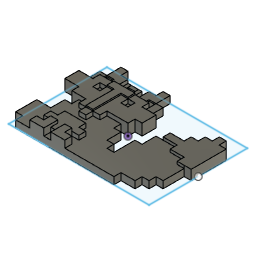
keychain (Autodesk Fusion 360 design; units mm, degrees)
Autodesk Fusion 360 part; units mm, degrees
note: some values were not read from the file. Set by a fixed rule: which sketch regions a step uses.
sketch "base" plane through (0, 0, 0) normal (0, 0, 1) x (1, 0, 0)
  line L0 (50, 0) -> (50, 35)
  line L1 (50, 35) -> (-50, 35)
  line L2 (-50, 35) -> (-50, -35)
  line L3 (-50, -35) -> (50, -35)
  line L4 (50, -35) -> (50, 0)
  dimension "d1" = 50
  dimension "d2" = 35
  dimension "d3" = 100
  dimension "d4" = 70
  dimension "d5" = 100
  dimension "d6" = 35
  constraint perpendicular L0 L1
  constraint perpendicular L1 L2
  constraint perpendicular L2 L3
  constraint perpendicular L1 L4
  measures "d1" distance of origin L0.start
  measures "d2" distance of L0.start L0.end
  measures "d3" distance of L0.end L1.end
  measures "d4" distance of L1.end L2.end
  measures "d5" distance of L2.end L3.end
  measures "d6" distance of L3.end L0.start
extrude "Extrude1" add sketch "base" along normal blind 10 makes body 1
sketch "fox" plane through (0, 0, 10) normal (0, 0, 1) x (-1, 0, 0)
  line L0 (-50, 35) -> (-50, -35)
  line L1 (-50, -35) -> (50, -35)
  line L2 (50, -35) -> (50, 35)
  line L3 (50, 35) -> (-50, 35)
  line L4 (40, -35) -> (40, -30)
  line L5 (45, -15) -> (50, -15)
  line L6 (50, -15) -> (50, -5)
  line L7 (50, -5) -> (40, -5)
  line L8 (40, -5) -> (40, 0)
  line L9 (40, 0) -> (35, 0)
  line L10 (35, 0) -> (35, 5)
  line L11 (35, 5) -> (40, 5)
  line L12 (40, 5) -> (40, 15)
  line L13 (40, 15) -> (50, 15)
  line L14 (50, 15) -> (50, 30)
  line L15 (50, 30) -> (45, 30)
  line L16 (45, 30) -> (45, 35)
  line L17 (45, 35) -> (-25, 35)
  line L18 (40, -35) -> (35, -35)
  line L19 (35, -35) -> (35, -30)
  line L20 (35, -30) -> (30, -30)
  line L21 (30, -30) -> (30, -20)
  line L22 (30, -20) -> (15, -20)
  line L23 (15, -20) -> (15, -25)
  line L24 (10, -35) -> (5, -35)
  line L25 (5, -35) -> (5, -25)
  line L26 (5, -25) -> (0, -25)
  line L27 (0, -25) -> (0, -15)
  line L28 (0, -15) -> (-5, -15)
  line L29 (-5, -15) -> (-5, -5)
  line L30 (-5, -5) -> (0, -5)
  line L31 (0, -5) -> (0, 0)
  line L32 (0, 0) -> (5, 0)
  line L33 (5, 0) -> (5, 5)
  line L34 (5, 5) -> (0, 5)
  line L35 (0, 5) -> (0, 15)
  line L36 (0, 15) -> (-5, 15)
  line L37 (-5, 15) -> (-5, 20)
  line L38 (-5, 20) -> (-10, 20)
  line L39 (-10, 20) -> (-10, 5)
  line L40 (-10, 5) -> (-15, 5)
  line L41 (-15, 5) -> (-15, -5)
  line L42 (-15, -5) -> (-20, -5)
  line L43 (-20, -5) -> (-20, -10)
  line L44 (-20, -10) -> (-30, -10)
  line L45 (-30, -10) -> (-30, -15)
  line L46 (-30, -15) -> (-35, -15)
  line L47 (-35, -15) -> (-35, -20)
  line L48 (-35, -20) -> (-40, -20)
  line L49 (-40, -20) -> (-40, -25)
  line L50 (-40, -25) -> (-45, -25)
  line L51 (-45, -25) -> (-45, -20)
  line L52 (-45, -20) -> (-50, -20)
  line L53 (-50, -20) -> (-50, 5)
  line L54 (-50, 5) -> (-45, 5)
  line L55 (-45, 5) -> (-45, 20)
  line L56 (-45, 20) -> (-40, 20)
  line L57 (-40, 20) -> (-40, 25)
  line L58 (-40, 25) -> (-35, 25)
  line L59 (-35, 25) -> (-35, 30)
  line L60 (-35, 30) -> (-25, 30)
  line L61 (-25, 30) -> (-25, 35)
  line L62 (40, -30) -> (40, -25)
  line L63 (40, -25) -> (45, -25)
  line L64 (45, -25) -> (45, -15)
  line L65 (10, -35) -> (10, -30)
  line L66 (10, -30) -> (15, -30)
  line L67 (15, -30) -> (15, -25)
  dimension "d9" = 5
  dimension "d12" = 5
  dimension "d14" = 10
  dimension "d15" = 10
  dimension "d16" = 5
  dimension "d17" = 5
  dimension "d18" = 5
  dimension "d19" = 5
  dimension "d20" = 10
  dimension "d21" = 10
  dimension "d22" = 15
  dimension "d23" = 5
  dimension "d24" = 5
  dimension "d25" = 70
  dimension "d26" = 5
  dimension "d27" = 5
  dimension "d28" = 5
  dimension "d29" = 10
  dimension "d30" = 15
  dimension "d31" = 5
  dimension "d34" = 5
  dimension "d35" = 10
  dimension "d36" = 5
  dimension "d37" = 10
  dimension "d38" = 5
  dimension "d39" = 10
  dimension "d40" = 5
  dimension "d41" = 5
  dimension "d42" = 5
  dimension "d43" = 5
  dimension "d44" = 5
  dimension "d45" = 10
  dimension "d46" = 5
  dimension "d47" = 5
  dimension "d48" = 5
  dimension "d49" = 15
  dimension "d50" = 5
  dimension "d51" = 10
  dimension "d52" = 5
  dimension "d53" = 5
  dimension "d54" = 10
  dimension "d55" = 5
  dimension "d56" = 5
  dimension "d57" = 5
  dimension "d58" = 5
  dimension "d59" = 5
  dimension "d60" = 5
  dimension "d61" = 5
  dimension "d62" = 5
  dimension "d63" = 25
  dimension "d64" = 5
  dimension "d65" = 15
  dimension "d66" = 5
  dimension "d67" = 5
  dimension "d68" = 5
  dimension "d69" = 5
  dimension "d70" = 10
  dimension "d71" = 5
  dimension "d78" = 5
  dimension "d79" = 5
  dimension "d152" = 5
  dimension "d153" = 5
  dimension "d154" = 5
  constraint coincident L1 L4.start
  constraint perpendicular L2 L5
  constraint perpendicular L5 L6
  constraint perpendicular L6 L7
  constraint perpendicular L7 L8
  constraint perpendicular L6 L9
  constraint perpendicular L9 L10
  constraint perpendicular L2 L11
  constraint perpendicular L7 L12
  constraint perpendicular L2 L13
  constraint perpendicular L13 L14
  constraint perpendicular L14 L15
  constraint perpendicular L3 L16
  constraint coincident L3 L17.end
  constraint perpendicular L16 L17
  constraint perpendicular L4 L18
  constraint perpendicular L18 L19
  constraint perpendicular L4 L20
  constraint perpendicular L18 L21
  constraint perpendicular L0 L22
  constraint perpendicular L22 L23
  constraint perpendicular L24 L25
  constraint perpendicular L25 L26
  constraint perpendicular L24 L27
  constraint perpendicular L27 L28
  constraint perpendicular L28 L29
  constraint perpendicular L23 L30
  constraint perpendicular L28 L31
  constraint perpendicular L23 L32
  constraint perpendicular L32 L33
  constraint perpendicular L33 L34
  constraint perpendicular L34 L35
  constraint perpendicular L35 L36
  constraint perpendicular L36 L37
  constraint perpendicular L37 L38
  constraint perpendicular L36 L39
  constraint perpendicular L39 L40
  constraint perpendicular L40 L41
  constraint perpendicular L41 L42
  constraint perpendicular L42 L43
  constraint perpendicular L41 L44
  constraint perpendicular L44 L45
  constraint perpendicular L25 L46
  constraint perpendicular L44 L47
  constraint perpendicular L25 L48
  constraint perpendicular L44 L49
  constraint perpendicular L25 L50
  constraint perpendicular L44 L51
  constraint perpendicular L0 L52
  constraint perpendicular L52 L53
  constraint perpendicular L53 L54
  constraint perpendicular L54 L55
  constraint perpendicular L55 L56
  constraint perpendicular L56 L57
  constraint perpendicular L55 L58
  constraint perpendicular L58 L59
  constraint perpendicular L55 L60
  constraint perpendicular L17 L61
  constraint parallel L4 L62
  constraint perpendicular L62 L63
  constraint perpendicular L5 L64
  constraint perpendicular L1 L65
  constraint perpendicular L65 L66
  constraint perpendicular L1 L67
  measures "d9" distance of L4.start L4.end
  measures "d12" distance of L5.start L5.end
  measures "d14" distance of L5.end L6.end
  measures "d15" distance of L6.end L7.end
  measures "d16" distance of L7.end L8.end
  measures "d17" distance of L8.end L9.end
  measures "d18" distance of L9.end L10.end
  measures "d19" distance of L10.end L11.end
  measures "d20" distance of L11.end L12.end
  measures "d21" distance of L12.end L13.end
  measures "d22" distance of L13.end L14.end
  measures "d23" distance of L14.end L15.end
  measures "d24" distance of L15.end L16.end
  measures "d25" distance of L16.end L17.end
  measures "d26" distance of L4.start L18.end
  measures "d27" distance of L18.end L19.end
  measures "d28" distance of L19.end L20.end
  measures "d29" distance of L20.end L21.end
  measures "d30" distance of L21.end L22.end
  measures "d31" distance of L22.end L23.end
  measures "d34" distance of L24.start L24.end
  measures "d35" distance of L24.end L25.end
  measures "d36" distance of L25.end L26.end
  measures "d37" distance of L26.end L27.end
  measures "d38" distance of L27.end L28.end
  measures "d39" distance of L28.end L29.end
  measures "d40" distance of L29.end L30.end
  measures "d41" distance of L30.end L31.end
  measures "d42" distance of L31.end L32.end
  measures "d43" distance of L32.end L33.end
  measures "d44" distance of L33.end L34.end
  measures "d45" distance of L34.end L35.end
  measures "d46" distance of L35.end L36.end
  measures "d47" distance of L36.end L37.end
  measures "d48" distance of L37.end L38.end
  measures "d49" distance of L38.end L39.end
  measures "d50" distance of L39.end L40.end
  measures "d51" distance of L40.end L41.end
  measures "d52" distance of L41.end L42.end
  measures "d53" distance of L42.end L43.end
  measures "d54" distance of L43.end L44.end
  measures "d55" distance of L44.end L45.end
  measures "d56" distance of L45.end L46.end
  measures "d57" distance of L46.end L47.end
  measures "d58" distance of L47.end L48.end
  measures "d59" distance of L48.end L49.end
  measures "d60" distance of L49.end L50.end
  measures "d61" distance of L50.end L51.end
  measures "d62" distance of L51.end L52.end
  measures "d63" distance of L52.end L53.end
  measures "d64" distance of L53.end L54.end
  measures "d65" distance of L54.end L55.end
  measures "d66" distance of L55.end L56.end
  measures "d67" distance of L56.end L57.end
  measures "d68" distance of L57.end L58.end
  measures "d69" distance of L58.end L59.end
  measures "d70" distance of L59.end L60.end
  measures "d71" distance of L60.end L17.end
  measures "d78" distance of L4.end L62.end
  measures "d79" distance of L62.end L63.end
  measures "d152" distance of L24.start L65.end
  measures "d153" distance of L65.end L66.end
  measures "d154" distance of L66.end L23.end
extrude "Extrude2" cut sketch "fox" against normal blind 0.1 contours L0 L1 L2 L3 L4 L5 L6 L7 L8 L9 L10 L11 L12 L13 L14 L15 L16 L17 L18 L19 L20 L21 L22 L23 L24 L25 L26 L27 L28 L29 L30 L31 L32 L33 L34 L35 L36 L37 L38 L39 L40 L41 L42 L43 L44 L45 L46 L47 L48 L49 L50 L51 L52 L53 L54 L55 L56 L57 L58 L59 L60 L61 L62 L63 L64 L65 L66 L67 bodies 1
extrude "Extrude3" add 1 faces at (-18.3333, 6.6667, 9.9) along direction (0, 0, 1) blind 0.1 on bodies 1 bodies 1
extrude "Extrude4" cut sketch "fox" against normal blind 10 contours L0 L3 L54 L55 L56 L57 L58 L59 L60 L61 | L0 L1 L25 L26 L27 L28 L29 L30 L31 L32 L33 L34 L35 L36 L37 L38 L39 L40 L41 L42 L43 L44 L45 L46 L47 L48 L49 L50 L51 L52 | L2 L3 L15 L16 | L1 L19 L20 L21 L22 L23 L65 L66 L67 | L2 L7 L8 L9 L10 L11 L12 L13 | L1 L2 L4 L5 L62 L63 L64 bodies 1
sketch "ears" plane through (0, 0, 10) normal (0, 0, 1) x (-1, 0, 0)
  line L0 (-45, 5) -> (-50, 5)
  line L1 (-50, 5) -> (-50, -20)
  line L2 (-50, -20) -> (-45, -20)
  line L3 (-45, -20) -> (-45, -25)
  line L4 (-45, -25) -> (-40, -25)
  line L5 (-40, -25) -> (-40, -20)
  line L6 (-40, -20) -> (-35, -20)
  line L7 (-35, -20) -> (-35, -15)
  line L8 (-35, -15) -> (-30, -15)
  line L9 (-30, -15) -> (-30, -10)
  line L10 (-30, -10) -> (-20, -10)
  line L11 (-20, -10) -> (-20, -5)
  line L12 (-20, -5) -> (-15, -5)
  line L13 (-15, -5) -> (-15, 5)
  line L14 (-15, 5) -> (-10, 5)
  line L15 (-10, 5) -> (-10, 20)
  line L16 (-10, 20) -> (-5, 20)
  line L17 (-5, 20) -> (-5, 15)
  line L18 (-5, 15) -> (0, 15)
  line L19 (0, 15) -> (0, 5)
  line L20 (0, 5) -> (5, 5)
  line L21 (5, 5) -> (5, 0)
  line L22 (5, 0) -> (0, 0)
  line L23 (0, 0) -> (0, -5)
  line L24 (0, -5) -> (-5, -5)
  line L25 (-5, -5) -> (-5, -15)
  line L26 (-5, -15) -> (0, -15)
  line L27 (0, -15) -> (0, -25)
  line L28 (0, -25) -> (5, -25)
  line L29 (5, -25) -> (5, -35)
  line L30 (5, -35) -> (10, -35)
  line L31 (40, -35) -> (40, -25)
  line L32 (45, -15) -> (50, -15)
  line L33 (50, -15) -> (50, -5)
  line L34 (50, -5) -> (40, -5)
  line L35 (40, -5) -> (40, 0)
  line L36 (40, 0) -> (35, 0)
  line L37 (35, 0) -> (35, 5)
  line L38 (35, 5) -> (40, 5)
  line L39 (40, 5) -> (40, 15)
  line L40 (40, 15) -> (50, 15)
  line L41 (50, 15) -> (50, 30)
  line L42 (50, 30) -> (45, 30)
  line L43 (45, 30) -> (45, 35)
  line L44 (45, 35) -> (-25, 35)
  line L45 (-25, 35) -> (-25, 30)
  line L46 (-25, 30) -> (-35, 30)
  line L47 (-35, 30) -> (-35, 25)
  line L48 (-35, 25) -> (-40, 25)
  line L49 (-40, 25) -> (-40, 20)
  line L50 (-40, 20) -> (-45, 20)
  line L51 (-45, 20) -> (-45, 5)
  line L52 (40, -25) -> (45, -25)
  line L53 (45, -25) -> (45, -15)
  line L54 (40, -25) -> (35, -25)
  line L55 (35, -25) -> (35, -20)
  line L56 (35, -20) -> (40, -20)
  line L57 (40, -20) -> (40, -25)
  line L58 (10, -25) -> (5, -25)
  line L59 (5, -25) -> (5, -20)
  line L60 (5, -20) -> (10, -20)
  line L61 (10, -20) -> (10, -25)
  line L62 (10, -35) -> (10, -30)
  line L63 (10, -30) -> (15, -30)
  line L64 (15, -30) -> (15, -20)
  line L65 (15, -20) -> (30, -20)
  line L66 (30, -20) -> (30, -30)
  line L67 (30, -30) -> (35, -30)
  line L68 (35, -30) -> (35, -35)
  line L69 (35, -35) -> (40, -35)
  dimension "d80" = 5
  dimension "d81" = 5
  dimension "d82" = 5
  dimension "d83" = 5
  dimension "d84" = 5
  dimension "d85" = 5
  dimension "d86" = 5
  dimension "d87" = 5
  constraint coincident L31.end L52.start
  constraint perpendicular L31 L54
  constraint perpendicular L52 L55
  constraint perpendicular L31 L56
  constraint perpendicular L52 L57
  constraint perpendicular L28 L59
  constraint perpendicular L29 L60
  constraint perpendicular L58 L61
  measures "d80" distance of L31.end L54.end
  measures "d81" distance of L54.end L55.end
  measures "d82" distance of L55.end L56.end
  measures "d83" distance of L56.end L31.end
  measures "d84" distance of L58.start L28.end
  measures "d85" distance of L28.end L59.end
  measures "d86" distance of L59.end L60.end
  measures "d87" distance of L60.end L58.start
sketch "eyes" plane through (0, 0, 10) normal (0, 0, 1) x (-1, 0, 0)
  line L0 (35, -15) -> (30, -15)
  line L1 (30, -15) -> (30, -10)
  line L2 (30, -10) -> (35, -10)
  line L3 (35, -10) -> (35, -15)
  line L4 (15, -15) -> (10, -15)
  line L5 (10, -15) -> (10, -10)
  line L6 (10, -10) -> (15, -10)
  line L7 (15, -10) -> (15, -15)
  dimension "d88" = 5
  dimension "d89" = 5
  dimension "d90" = 5
  dimension "d91" = 5
  dimension "d92" = 5
  dimension "d93" = 5
  dimension "d94" = 5
  dimension "d95" = 5
  constraint horizontal L0
  constraint perpendicular L0 L1
  constraint perpendicular L1 L2
  constraint perpendicular L2 L3
  constraint perpendicular L1 L4
  constraint perpendicular L0 L5
  constraint perpendicular L1 L6
  constraint perpendicular L0 L7
  measures "d88" distance of L0.start L0.end
  measures "d89" distance of L0.end L1.end
  measures "d90" distance of L1.end L2.end
  measures "d91" distance of L2.end L0.start
  measures "d92" distance of L4.start L4.end
  measures "d93" distance of L4.end L5.end
  measures "d94" distance of L5.end L6.end
  measures "d95" distance of L6.end L4.start
sketch "face" plane through (0, 0, 10) normal (0, 0, 1) x (-1, 0, 0)
  line L0 (35, 0) -> (30, 0)
  line L1 (30, 0) -> (30, 5)
  line L2 (30, 5) -> (25, 5)
  line L3 (20, 5) -> (15, 5)
  line L4 (15, 5) -> (15, 0)
  line L5 (15, 0) -> (10, 0)
  line L6 (10, 0) -> (0, 0)
  line L7 (0, 0) -> (0, -5)
  line L8 (0, -5) -> (-5, -5)
  line L9 (-5, -5) -> (-5, -15)
  line L10 (-5, -15) -> (5, -15)
  line L11 (5, -15) -> (5, -20)
  line L12 (5, -20) -> (10, -20)
  line L13 (10, -20) -> (15, -20)
  line L14 (15, -20) -> (15, -15)
  line L15 (30, -15) -> (30, -20)
  line L16 (30, -20) -> (40, -20)
  line L17 (40, -20) -> (40, -15)
  line L18 (40, -15) -> (50, -15)
  line L19 (50, -15) -> (50, -5)
  line L20 (50, -5) -> (40, -5)
  line L21 (40, -5) -> (40, 0)
  line L22 (40, 0) -> (35, 0)
  line L23 (30, -15) -> (25, -15)
  line L24 (25, -15) -> (25, 5)
  line L25 (15, -15) -> (20, -15)
  line L26 (20, -15) -> (20, 5)
  dimension "d96" = 5
  dimension "d97" = 5
  dimension "d98" = 5
  dimension "d102" = 5
  dimension "d103" = 5
  dimension "d104" = 5
  dimension "d105" = 10
  dimension "d106" = 5
  dimension "d107" = 5
  dimension "d108" = 10
  dimension "d109" = 5
  dimension "d110" = 5
  dimension "d111" = 5
  dimension "d112" = 5
  dimension "d113" = 5
  dimension "d114" = 10
  dimension "d115" = 5
  dimension "d116" = 10
  dimension "d117" = 10
  dimension "d118" = 10
  dimension "d119" = 5
  dimension "d120" = 5
  dimension "d121" = 5
  dimension "d122" = 20
  dimension "d123" = 5
  dimension "d124" = 20
  constraint horizontal L0
  constraint perpendicular L0 L1
  constraint perpendicular L1 L2
  constraint perpendicular L3 L4
  constraint perpendicular L4 L5
  constraint parallel L5 L6
  constraint perpendicular L5 L7
  constraint perpendicular L7 L8
  constraint perpendicular L5 L9
  constraint perpendicular L9 L10
  constraint perpendicular L10 L11
  constraint perpendicular L9 L12
  constraint parallel L12 L13
  constraint perpendicular L12 L14
  constraint perpendicular L12 L15
  constraint perpendicular L15 L16
  constraint perpendicular L12 L17
  constraint perpendicular L17 L18
  constraint perpendicular L12 L19
  constraint perpendicular L19 L20
  constraint perpendicular L12 L21
  constraint perpendicular L21 L22
  constraint perpendicular L15 L23
  constraint perpendicular L2 L24
  constraint perpendicular L14 L25
  constraint perpendicular L25 L26
  measures "d96" distance of L0.start L0.end
  measures "d97" distance of L0.end L1.end
  measures "d98" distance of L1.end L2.end
  measures "d102" distance of L3.start L3.end
  measures "d103" distance of L3.end L4.end
  measures "d104" distance of L4.end L5.end
  measures "d105" distance of L5.end L6.end
  measures "d106" distance of L6.end L7.end
  measures "d107" distance of L7.end L8.end
  measures "d108" distance of L9.end L10.end
  measures "d109" distance of L10.end L11.end
  measures "d110" distance of L11.end L12.end
  measures "d111" distance of L12.end L13.end
  measures "d112" distance of L13.end L14.end
  measures "d113" distance of L15.start L15.end
  measures "d114" distance of L15.end L16.end
  measures "d115" distance of L16.end L17.end
  measures "d116" distance of L17.end L18.end
  measures "d117" distance of L18.end L19.end
  measures "d118" distance of L19.end L20.end
  measures "d119" distance of L20.end L21.end
  measures "d120" distance of L21.end L0.start
  measures "d121" distance of L15.start L23.end
  measures "d122" distance of L23.end L2.end
  measures "d123" distance of L14.end L25.end
  measures "d124" distance of L25.end L3.start
sketch "nose" plane through (0, 0, 10) normal (0, 0, 1) x (-1, 0, 0)
  line L0 (25, 5) -> (20, 5)
  line L1 (20, 5) -> (20, 10)
  line L2 (20, 10) -> (25, 10)
  line L3 (25, 10) -> (25, 5)
  dimension "d125" = 5
  dimension "d126" = 5
  constraint horizontal L0
  constraint vertical L1
  constraint horizontal L2
  constraint vertical L3
  measures "d125" distance of L0.start L0.end
  measures "d126" distance of L0.start L2.end
sketch "chest" plane through (0, 0, 10) normal (0, 0, 1) x (-1, 0, 0)
  line L0 (25, 30) -> (20, 30)
  line L1 (20, 30) -> (20, 25)
  line L2 (20, 25) -> (10, 25)
  line L3 (10, 25) -> (10, 20)
  line L4 (10, 20) -> (15, 20)
  line L5 (15, 20) -> (15, 15)
  line L6 (15, 15) -> (30, 15)
  line L7 (30, 15) -> (30, 20)
  line L8 (30, 20) -> (35, 20)
  line L9 (35, 20) -> (35, 25)
  line L10 (35, 25) -> (25, 25)
  line L11 (25, 25) -> (25, 30)
  dimension "d127" = 5
  dimension "d128" = 5
  dimension "d129" = 10
  dimension "d130" = 5
  dimension "d131" = 5
  dimension "d132" = 5
  dimension "d133" = 15
  dimension "d134" = 5
  dimension "d135" = 5
  dimension "d136" = 5
  dimension "d137" = 10
  dimension "d138" = 5
  constraint horizontal L0
  constraint perpendicular L0 L1
  constraint perpendicular L1 L2
  constraint perpendicular L2 L3
  constraint perpendicular L3 L4
  constraint perpendicular L4 L5
  constraint perpendicular L5 L6
  constraint perpendicular L6 L7
  constraint perpendicular L5 L8
  constraint perpendicular L6 L9
  constraint perpendicular L5 L10
  constraint perpendicular L10 L11
  measures "d127" distance of L0.start L0.end
  measures "d128" distance of L0.end L1.end
  measures "d129" distance of L1.end L2.end
  measures "d130" distance of L2.end L3.end
  measures "d131" distance of L3.end L4.end
  measures "d132" distance of L4.end L5.end
  measures "d133" distance of L5.end L6.end
  measures "d134" distance of L6.end L7.end
  measures "d135" distance of L7.end L8.end
  measures "d136" distance of L8.end L9.end
  measures "d137" distance of L9.end L10.end
  measures "d138" distance of L10.end L0.start
sketch "legs" plane through (0, 0, 10) normal (0, 0, 1) x (-1, 0, 0)
  line L0 (25, 30) -> (25, 35)
  line L1 (25, 35) -> (35, 35)
  line L2 (35, 35) -> (35, 30)
  line L3 (35, 30) -> (30, 30)
  line L4 (30, 30) -> (30, 25)
  line L5 (30, 25) -> (25, 25)
  line L6 (25, 25) -> (25, 30)
  line L7 (20, 25) -> (20, 35)
  line L8 (20, 35) -> (10, 35)
  line L9 (10, 35) -> (10, 30)
  line L10 (10, 30) -> (15, 30)
  line L11 (15, 30) -> (15, 25)
  line L12 (15, 25) -> (20, 25)
  dimension "d139" = 5
  dimension "d140" = 10
  dimension "d141" = 5
  dimension "d142" = 5
  dimension "d143" = 5
  dimension "d144" = 5
  dimension "d145" = 5
  dimension "d146" = 10
  dimension "d147" = 10
  dimension "d148" = 5
  dimension "d149" = 5
  dimension "d150" = 5
  dimension "d151" = 5
  constraint vertical L0
  constraint perpendicular L0 L1
  constraint perpendicular L1 L2
  constraint perpendicular L2 L3
  constraint perpendicular L3 L4
  constraint perpendicular L4 L5
  constraint perpendicular L5 L6
  constraint vertical L7
  constraint perpendicular L7 L8
  constraint perpendicular L8 L9
  constraint perpendicular L9 L10
  constraint perpendicular L10 L11
  constraint perpendicular L11 L12
  measures "d139" distance of L0.start L0.end
  measures "d140" distance of L0.end L1.end
  measures "d141" distance of L1.end L2.end
  measures "d142" distance of L2.end L3.end
  measures "d143" distance of L3.end L4.end
  measures "d144" distance of L4.end L5.end
  measures "d145" distance of L5.end L0.start
  measures "d146" distance of L7.start L7.end
  measures "d147" distance of L7.end L8.end
  measures "d148" distance of L8.end L9.end
  measures "d149" distance of L9.end L10.end
  measures "d150" distance of L10.end L11.end
  measures "d151" distance of L11.end L7.start
sketch "tail" plane through (0, 0, 10) normal (0, 0, 1) x (-1, 0, 0)
  line L0 (-45, 5) -> (-50, 5)
  line L1 (-50, 5) -> (-50, -20)
  line L2 (-50, -20) -> (-45, -20)
  line L3 (-45, -20) -> (-45, -25)
  line L4 (-45, -25) -> (-40, -25)
  line L5 (-40, -25) -> (-40, -20)
  line L6 (-40, -20) -> (-35, -20)
  line L7 (-35, -20) -> (-35, -15)
  line L8 (-35, -15) -> (-30, -15)
  line L9 (-30, -15) -> (-30, -10)
  line L10 (-30, -10) -> (-25, -10)
  line L11 (-25, -10) -> (-20, -10)
  line L12 (-20, -10) -> (-20, -5)
  line L13 (-20, -5) -> (-25, -5)
  line L14 (-25, -5) -> (-30, -5)
  line L15 (-30, -5) -> (-30, 0)
  line L16 (-30, 0) -> (-40, 0)
  line L17 (-40, 0) -> (-40, 5)
  line L18 (-40, 5) -> (-45, 5)
  dimension "d162" = 5
  dimension "d163" = 25
  dimension "d164" = 5
  dimension "d165" = 5
  dimension "d166" = 5
  dimension "d167" = 5
  dimension "d168" = 5
  dimension "d169" = 5
  dimension "d170" = 5
  dimension "d173" = 5
  dimension "d174" = 5
  dimension "d175" = 5
  dimension "d176" = 5
  dimension "d177" = 5
  dimension "d178" = 5
  dimension "d179" = 10
  dimension "d180" = 5
  dimension "d181" = 5
  constraint perpendicular L0 L1
  constraint perpendicular L1 L2
  constraint perpendicular L2 L3
  constraint perpendicular L1 L4
  constraint perpendicular L4 L5
  constraint perpendicular L1 L6
  constraint perpendicular L6 L7
  constraint perpendicular L1 L8
  constraint perpendicular L8 L9
  constraint perpendicular L9 L10
  constraint perpendicular L9 L11
  constraint perpendicular L10 L12
  constraint perpendicular L9 L13
  constraint perpendicular L9 L14
  constraint perpendicular L10 L15
  constraint perpendicular L9 L16
  constraint perpendicular L10 L17
  constraint perpendicular L9 L18
  measures "d162" distance of L0.start L0.end
  measures "d163" distance of L0.end L1.end
  measures "d164" distance of L1.end L2.end
  measures "d165" distance of L2.end L3.end
  measures "d166" distance of L3.end L4.end
  measures "d167" distance of L5.end L6.end
  measures "d168" distance of L6.end L7.end
  measures "d169" distance of L7.end L8.end
  measures "d170" distance of L8.end L9.end
  measures "d173" distance of L9.end L10.end
  measures "d174" distance of L10.end L11.end
  measures "d175" distance of L11.end L12.end
  measures "d176" distance of L12.end L13.end
  measures "d177" distance of L13.end L14.end
  measures "d178" distance of L14.end L15.end
  measures "d179" distance of L15.end L16.end
  measures "d180" distance of L16.end L17.end
  measures "d181" distance of L17.end L0.start
extrude "Extrude5" cut sketch "chest" against normal blind 1 bodies 1
extrude "Extrude6" cut sketch "face" against normal blind 2 bodies 1
extrude "Extrude7" cut sketch "eyes" sketch "ears" against normal blind 5 of sketch 2 contours L58 L59 L60 L61 | L54 L55 L56 L57 bodies 1
extrude "Extrude8" cut sketch "nose" against normal blind 5 bodies 1
extrude "Extrude9" cut sketch "tail" against normal blind 2 bodies 1
sketch "contour " plane through (0, 0, 10) normal (0, 0, 1) x (-1, 0, 0)
  line L0 (-45, 5) -> (-45, 20)
  line L1 (-45, 20) -> (-40, 20)
  line L2 (-40, 20) -> (-40, 25)
  line L3 (-40, 25) -> (-35, 25)
  line L4 (-35, 25) -> (-35, 30)
  line L5 (-35, 30) -> (-25, 30)
  line L6 (-25, 30) -> (-25, 35)
  line L7 (-25, 35) -> (10, 35)
  line L8 (10, 35) -> (10, 30)
  line L9 (10, 30) -> (15, 30)
  line L10 (15, 30) -> (15, 25)
  line L11 (15, 25) -> (10, 25)
  line L12 (10, 25) -> (10, 20)
  line L13 (10, 20) -> (15, 20)
  line L14 (15, 20) -> (15, 15)
  line L15 (15, 15) -> (30, 15)
  line L16 (30, 15) -> (30, 20)
  line L17 (30, 20) -> (35, 20)
  line L18 (35, 20) -> (35, 25)
  line L19 (35, 25) -> (30, 25)
  line L20 (30, 25) -> (30, 30)
  line L21 (30, 30) -> (35, 30)
  line L22 (35, 30) -> (35, 35)
  line L23 (35, 35) -> (45, 35)
  line L24 (45, 35) -> (45, 30)
  line L25 (45, 30) -> (50, 30)
  line L26 (50, 30) -> (50, 15)
  line L27 (50, 15) -> (40, 15)
  line L28 (40, 15) -> (40, 5)
  line L29 (40, 5) -> (35, 5)
  line L30 (35, 5) -> (35, 0)
  line L31 (35, 0) -> (30, 0)
  line L32 (30, 0) -> (30, 5)
  line L33 (30, 5) -> (25, 5)
  line L34 (25, 5) -> (25, 10)
  line L35 (25, 10) -> (20, 10)
  line L36 (20, 10) -> (20, 5)
  line L37 (20, 5) -> (15, 5)
  line L38 (15, 5) -> (15, 0)
  line L39 (15, 0) -> (5, 0)
  line L40 (5, 0) -> (5, 5)
  line L41 (5, 5) -> (0, 5)
  line L42 (0, 5) -> (0, 15)
  line L43 (0, 15) -> (-5, 15)
  line L44 (-5, 15) -> (-5, 20)
  line L45 (-5, 20) -> (-10, 20)
  line L46 (-10, 20) -> (-10, 5)
  line L47 (-10, 5) -> (-15, 5)
  line L48 (-15, 5) -> (-15, -5)
  line L49 (-15, -5) -> (-30, -5)
  line L50 (-30, -5) -> (-30, 0)
  line L51 (-30, 0) -> (-40, 0)
  line L52 (-40, 0) -> (-40, 5)
  line L53 (-40, 5) -> (-45, 5)
  line L54 (45, -15) -> (40, -15)
  line L55 (40, -15) -> (40, -25)
  line L56 (40, -25) -> (45, -25)
  line L57 (45, -25) -> (45, -15)
  line L58 (30, -20) -> (30, -30)
  line L59 (30, -30) -> (35, -30)
  line L60 (35, -30) -> (35, -35)
  line L61 (35, -35) -> (40, -35)
  line L62 (40, -35) -> (40, -25)
  line L63 (35, -25) -> (40, -25)
  line L64 (35, -25) -> (35, -20)
  line L65 (35, -20) -> (30, -20)
  line L66 (15, -20) -> (10, -20)
  line L67 (10, -20) -> (10, -25)
  line L68 (10, -25) -> (5, -25)
  line L69 (5, -25) -> (5, -35)
  line L70 (5, -35) -> (10, -35)
  line L71 (10, -35) -> (10, -30)
  line L72 (10, -30) -> (15, -30)
  line L73 (15, -30) -> (15, -20)
  line L74 (5, -25) -> (0, -25)
  line L75 (0, -25) -> (0, -15)
  line L76 (0, -15) -> (5, -15)
  line L77 (5, -15) -> (5, -25)
  line L78 (25, 30) -> (20, 30)
  line L79 (20, 30) -> (20, 35)
  line L80 (20, 35) -> (25, 35)
  line L81 (25, 35) -> (25, 30)
  dimension "d192" = 15
  constraint vertical L0
  constraint perpendicular L0 L1
  constraint perpendicular L1 L2
  constraint perpendicular L2 L3
  constraint perpendicular L3 L4
  constraint perpendicular L4 L5
  constraint perpendicular L5 L6
  constraint perpendicular L6 L7
  constraint perpendicular L7 L8
  constraint perpendicular L8 L9
  constraint perpendicular L9 L10
  constraint perpendicular L10 L11
  constraint perpendicular L11 L12
  constraint perpendicular L12 L13
  constraint perpendicular L13 L14
  constraint perpendicular L14 L15
  constraint perpendicular L15 L16
  constraint perpendicular L16 L17
  constraint perpendicular L17 L18
  constraint perpendicular L18 L19
  constraint perpendicular L17 L20
  constraint perpendicular L18 L21
  constraint perpendicular L17 L22
  constraint perpendicular L22 L23
  constraint perpendicular L23 L24
  constraint perpendicular L24 L25
  constraint perpendicular L25 L26
  constraint perpendicular L26 L27
  constraint perpendicular L27 L28
  constraint perpendicular L26 L29
  constraint perpendicular L29 L30
  constraint perpendicular L30 L31
  constraint perpendicular L29 L32
  constraint perpendicular L32 L33
  constraint perpendicular L33 L34
  constraint perpendicular L34 L35
  constraint perpendicular L35 L36
  constraint perpendicular L36 L37
  constraint perpendicular L37 L38
  constraint perpendicular L38 L39
  constraint perpendicular L39 L40
  constraint perpendicular L40 L41
  constraint perpendicular L41 L42
  constraint perpendicular L42 L43
  constraint perpendicular L43 L44
  constraint perpendicular L44 L45
  constraint perpendicular L45 L46
  constraint perpendicular L44 L47
  constraint perpendicular L45 L48
  constraint perpendicular L48 L49
  constraint perpendicular L49 L50
  constraint perpendicular L50 L51
  constraint perpendicular L51 L52
  constraint horizontal L54
  constraint perpendicular L54 L55
  constraint perpendicular L55 L56
  constraint perpendicular L54 L57
  constraint perpendicular L54 L58
  constraint perpendicular L58 L59
  constraint perpendicular L59 L60
  constraint perpendicular L60 L61
  constraint perpendicular L56 L62
  constraint perpendicular L62 L63
  constraint perpendicular L63 L64
  constraint perpendicular L58 L65
  constraint horizontal L66
  constraint perpendicular L66 L67
  constraint perpendicular L67 L68
  constraint perpendicular L66 L69
  constraint perpendicular L69 L70
  constraint perpendicular L70 L71
  constraint perpendicular L71 L72
  constraint perpendicular L66 L73
  constraint perpendicular L69 L74
  constraint perpendicular L74 L75
  constraint perpendicular L75 L76
  constraint perpendicular L68 L77
  constraint horizontal L78
  constraint vertical L79
  constraint horizontal L80
  constraint vertical L81
  measures "d192" distance of L0.start L0.end
extrude "Extrude10" add sketch "eyes" sketch "ears" against normal blind 4 separate body of sketch 2 contours L58 L59 L60 L61 | L54 L55 L56 L57 makes body 2 at (-6.6667, 21.6667, 10) makes body 3 at (-33.3333, 13.3333, 10) makes body 4 at (-13.3333, 13.3333, 10) makes body 5 at (-38.3333, 23.3333, 10)
extrude "Extrude11" cut 4 faces at (-33.3333, 13.3333, 10) (-13.3333, 13.3333, 10) (-6.6667, 21.6667, 10) (-38.3333, 23.3333, 10) along direction (0, 0, -1) blind 3 on bodies 2 3 4 5 bodies 2 3 4 5
extrude "Extrude12" cut sketch "legs" against normal blind 9 bodies 1
extrude "Extrude13" add 1 faces at (-23.3333, -6.6667, 5) along direction (0, 0, 1) blind 4 on bodies 1 bodies 1
extrude "Extrude14" cut sketch "contour " against normal blind 5 bodies 1
extrude "Extrude15" add 2 faces at (-26.6667, -30, 1) (-15, -33.3333, 1) along direction (0, 0, 1) blind 9 on bodies 1 bodies 1
extrude "Extrude16" cut 1 faces at (46.6667, 5, 8) along direction (0, 0, -1) blind 1 on bodies 1 bodies 1
extrude "Extrude17" cut 2 faces at (-38.3333, 23.3333, 7) (-6.6667, 21.6667, 7) along direction (0, 0, -1) blind 3 on bodies 2 5 bodies 1 2 5
extrude "Extrude18" cut 2 faces at (-33.3333, 13.3333, 7) (-13.3333, 13.3333, 7) along direction (0, 0, -1) blind 2 on bodies 3 4 bodies 3 4
extrude "Extrude19" cut 1 faces at (-23.3333, -6.6667, 9) along direction (0, 0, -1) blind 1 on bodies 1 bodies 1
extrude "Extrude20" cut 1 faces at (-23.3333, 18.3333, 10) along direction (0, 0, -1) blind 1 on bodies 1 bodies 1
extrude "Extrude21" cut 1 faces at (-23.3333, -18.3333, 9) along direction (0, 0, -1) blind 1 on bodies 1 bodies 1
sketch "chain1" plane through (0, 20, 0) normal (0, 1, 0) x (-1, 0, 0)
  line L0 (30, 9) -> (15, 9)
  line L1 (15, 9) -> (15, 8)
  line L2 (15, 8) -> (5, 8)
  line L3 (5, 8) -> (5, 5)
  line L4 (5, 5) -> (5, 4)
  line L5 (5, 4) -> (10, 4)
  line L6 (10, 4) -> (10, 5)
  line L7 (10, 5) -> (15, 5)
  line L8 (15, 5) -> (15, 0)
  line L9 (15, 0) -> (30, 0)
  line L10 (30, 0) -> (30, 5)
  line L11 (30, 5) -> (35, 5)
  line L12 (35, 5) -> (35, 4)
  line L13 (35, 4) -> (40, 4)
  line L14 (40, 4) -> (40, 5)
  line L15 (40, 5) -> (40, 8)
  line L16 (40, 8) -> (30, 8)
  line L17 (30, 8) -> (30, 9)
  line L18 (17.5, 5) -> (20, 5)
  line L19 (20, 5) -> (20, 2.5)
  line L20 (20, 2.5) -> (17.5, 2.5)
  line L21 (17.5, 2.5) -> (17.5, 5)
  line L22 (25, 5) -> (27.5, 5)
  line L23 (27.5, 5) -> (27.5, 2.5)
  line L24 (27.5, 2.5) -> (25, 2.5)
  line L25 (25, 2.5) -> (25, 5)
  constraint horizontal L18
  constraint perpendicular L18 L19
  constraint perpendicular L19 L20
  constraint perpendicular L18 L21
  constraint horizontal L22
  constraint vertical L23
  constraint horizontal L24
  constraint vertical L25
extrude "Extrude22" add sketch "chain1" along normal blind 7.5 contours L18 L19 L20 L21 | L22 L23 L24 L25 bodies 2 1 3 4 5
sketch "chain2" plane through (-20, 0, 0) normal (-1, 0, 0) x (0, -1, 0)
  line L0 (-20, 2.5) -> (-20, 5)
  line L1 (-20, 5) -> (-27.5, 5)
  line L2 (-27.5, 5) -> (-27.5, 2.5)
  line L3 (-27.5, 2.5) -> (-20, 2.5)
  line L4 (-27.5, 5) -> (-25, 5)
  line L5 (-25, 5) -> (-25, 2.5)
  line L6 (-25, 2.5) -> (-27.5, 2.5)
  line L7 (-27.5, 2.5) -> (-27.5, 5)
  constraint horizontal L4
  constraint vertical L5
  constraint horizontal L6
  constraint vertical L7
  constraint coincident L3 L5.end
  constraint coincident L1.end L2.start
extrude "Extrude23" add sketch "chain2" along normal blind 5 separate body contours L1 L2 L3 L4 L5 L6 L7 makes body 6
